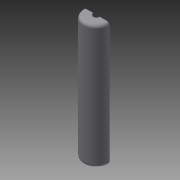
# Autodesk Inventor part: Wagon Hand Handle V04
Saved by Autodesk Inventor 2014 (Build 180170000, 170)
## iProperties
Created: 2013-11-30
Part Number: Wagon Hand Handle V04
Material: Generic
Document SubType Name: Modeling
Designer: steele
Density: 1 g/cm^3
Appearance: Default
Author: steele
Autodesk Inventor part; units mm, degrees
ref_plane "YZ Plane" through (0, 0, 0) normal (1, 0, 0) x (0, 1, 0)
ref_plane "XZ Plane" through (0, 0, 0) normal (0, 1, 0) x (-1, 0, 0)
ref_plane "XY Plane" through (0, 0, 0) normal (0, 0, 1) x (1, 0, 0)
sketch "Sketch1" plane through (0, 0, 0) normal (0, 0, 1) x (1, 0, 0)
  circle A0 centre (0, 0) radius 12.7
  circle A1 centre (0, 0) radius 3.302
  dimension "d0" = 25.4
  dimension "d1" = 6.604
  constraints: 2 centre point, 2 coincident
  measures "d0" diameter of A0
  measures "d1" diameter of A1
extrude "Extrusion1" add sketch "Sketch1" along normal mid plane 120.65
fillet "Fillet1" radius 3 2 edges at (-12.7, 0, 60.325) (-12.7, 0, -60.325)
sketch "Sketch3" plane through (0, 0, 60.325) normal (0, 0, 1) x (1, 0, 0)
  line L0 (-31, 0) -> (39, 0)
  line L1 (39, 0) -> (17, 30)
  line L2 (17, 30) -> (-16, 29)
  line L3 (-16, 29) -> (-31, 0)
  constraints: 8 end point, 1 horizontal
extrude "Extrusion2" cut sketch "Sketch3" against normal through all
sketch "Sketch4" plane through (-9.7, 0, 60.325) normal (0, 1, 0) x (1, 0, 0)
  line L0 (-3, 3) -> (-3, 117.65) projected
  line L1 (9.7, 0) -> (9.7, 120.65) construction
  circle A0 centre (9.7, 25.4) radius 8.8265
  circle A1 centre (9.7, 60.325) radius 8.8265
  circle A2 centre (9.7, 95.25) radius 8.8265
  circle A3 centre (9.7, 25.4) radius 5.7531
  circle A4 centre (9.7, 95.25) radius 5.7531
  circle A5 centre (9.7, 60.325) radius 5.7531
  line L2 (6.398, 120.65) -> (13.002, 120.65) projected
  dimension "d7" = 17.653
  dimension "d8" = 11.5062
  dimension "d16" = 60.325
  dimension "d17" = 25.4
  dimension "d18" = 25.4
  constraints: 6 centre point, 4 coincident, 4 equal radius, 2 end point, 2 point on line, 1 parallel
  measures "d7" diameter of A0
  measures "d8" diameter of A3
  measures "d16" distance of point (9.7, 60.325) L1.start
  measures "d17" distance of A0.centre L1.start
  measures "d18" distance from line of A2.centre L2
extrude "Extrusion3" cut sketch "Sketch4" against normal blind 9
sketch "Sketch7" plane through (-9.7, 0, 60.325) normal (0, 1, 0) x (1, 0, 0)
  line L0 (6.398, 52.1394) -> (6.398, 33.5856) projected
  line L1 (3.398, 34.5856) -> (3.398, 51.1394) construction
  line L2 (3.398, 34.2503) -> (3.398, 33.8516)
  line L3 (3.398, 33.8516) -> (1.9296, 33.8516)
  line L4 (1.9296, 33.8516) -> (1.9296, 32.4707)
  line L5 (1.9296, 32.4707) -> (3.398, 32.4707)
  line L6 (3.398, 32.4707) -> (3.398, 32.072)
  line L7 (3.398, 32.072) -> (0.398, 32.072)
  line L8 (0.398, 32.072) -> (0.398, 32.4707)
  line L9 (0.398, 32.4707) -> (1.5747, 32.4707)
  line L10 (1.5747, 32.4707) -> (1.5747, 33.8516)
  line L11 (1.5747, 33.8516) -> (0.398, 33.8516)
  line L12 (0.398, 33.8516) -> (0.398, 34.2503)
  line L13 (0.398, 34.2503) -> (3.398, 34.2503)
  spline S0 degree 2 poles (3.1598, 36.0833) (3.1938, 36.0371) (3.3153, 35.8815) (3.3518, 35.8086) knots 0 0 0 1 2 2 2
  spline S1 degree 2 poles (3.3518, 35.8086) (3.4053, 35.7089) (3.4612, 35.5217) (3.4612, 35.3516) knots 0 0 0 1 2 2 2
  spline S2 degree 2 poles (3.4612, 35.3516) (3.4612, 35.213) (3.3567, 34.9626) (3.2619, 34.8678) knots 0 0 0 1 2 2 2
  spline S3 degree 2 poles (3.2619, 34.8678) (3.1695, 34.7778) (2.8972, 34.6684) (2.7465, 34.6684) knots 0 0 0 1 2 2 2
  spline S4 degree 2 poles (2.7465, 34.6684) (2.5131, 34.6684) (2.1824, 34.8653) (2.0876, 35.0793) knots 0 0 0 1 2 2 2
  spline S5 degree 2 poles (2.0876, 35.0793) (2.0001, 35.2689) (1.9345, 35.7843) (1.9174, 36.0833) knots 0 0 0 1 2 2 2
  line L14 (1.9174, 36.0833) -> (1.8445, 36.0833)
  spline S6 degree 2 poles (1.8445, 36.0833) (1.7132, 36.0833) (1.5504, 36.0031) (1.5042, 35.9302) knots 0 0 0 1 2 2 2
  spline S7 degree 2 poles (1.5042, 35.9302) (1.458, 35.8572) (1.4288, 35.6482) (1.4288, 35.5363) knots 0 0 0 1 2 2 2
  spline S8 degree 2 poles (1.4288, 35.5363) (1.4288, 35.405) (1.5066, 35.0501) (1.582, 34.8726) knots 0 0 0 1 2 2 2
  line L15 (1.582, 34.8726) -> (1.582, 34.8507)
  line L16 (1.582, 34.8507) -> (1.1954, 34.8507)
  spline S9 degree 2 poles (1.1954, 34.8507) (1.1662, 34.9553) (1.0933, 35.3467) (1.0933, 35.5388) knots 0 0 0 1 2 2 2
  spline S10 degree 2 poles (1.0933, 35.5388) (1.0933, 35.7721) (1.1662, 36.0906) (1.261, 36.217) knots 0 0 0 1 2 2 2
  spline S11 degree 2 poles (1.261, 36.217) (1.3534, 36.341) (1.6476, 36.4626) (1.8591, 36.4626) knots 0 0 0 1 2 2 2
  line L17 (1.8591, 36.4626) -> (3.398, 36.4626)
  line L18 (3.398, 36.4626) -> (3.398, 36.0833)
  line L19 (3.398, 36.0833) -> (3.1598, 36.0833)
  line L20 (2.8437, 36.0833) -> (2.2189, 36.0833)
  spline S12 degree 2 poles (2.2189, 36.0833) (2.2311, 35.9472) (2.2724, 35.5363) (2.3113, 35.4075) knots 0 0 0 1 2 2 2
  spline S13 degree 2 poles (2.3113, 35.4075) (2.3575, 35.2567) (2.5495, 35.0598) (2.7197, 35.0598) knots 0 0 0 1 2 2 2
  spline S14 degree 2 poles (2.7197, 35.0598) (2.9142, 35.0598) (3.1111, 35.2786) (3.1111, 35.4877) knots 0 0 0 1 2 2 2
  spline S15 degree 2 poles (3.1111, 35.4877) (3.1111, 35.6652) (2.958, 35.9569) (2.8437, 36.0833) knots 0 0 0 1 2 2 2
  line L21 (3.398, 38.7624) -> (3.398, 38.3832)
  line L22 (3.398, 38.3832) -> (2.1144, 38.3832)
  spline S16 degree 2 poles (2.1144, 38.3832) (1.9588, 38.3832) (1.6914, 38.354) (1.6111, 38.3102) knots 0 0 0 1 2 2 2
  spline S17 degree 2 poles (1.6111, 38.3102) (1.526, 38.264) (1.4434, 38.0987) (1.4434, 37.9577) knots 0 0 0 1 2 2 2
  spline S18 degree 2 poles (1.4434, 37.9577) (1.4434, 37.8167) (1.5941, 37.5177) (1.7157, 37.3742) knots 0 0 0 1 2 2 2
  line L23 (1.7157, 37.3742) -> (3.398, 37.3742)
  line L24 (3.398, 37.3742) -> (3.398, 36.995)
  line L25 (3.398, 36.995) -> (1.1468, 36.995)
  line L26 (1.1468, 36.995) -> (1.1468, 37.3742)
  line L27 (1.1468, 37.3742) -> (1.3972, 37.3742)
  spline S19 degree 2 poles (1.3972, 37.3742) (1.244, 37.5444) (1.0836, 37.8726) (1.0836, 38.0574) knots 0 0 0 1 2 2 2
  spline S20 degree 2 poles (1.0836, 38.0574) (1.0836, 38.388) (1.5212, 38.7624) (1.9369, 38.7624) knots 0 0 0 1 2 2 2
  line L28 (1.9369, 38.7624) -> (3.398, 38.7624)
  line L29 (3.398, 41.0258) -> (3.398, 40.6465)
  line L30 (3.398, 40.6465) -> (3.1695, 40.6465)
  spline S21 degree 2 poles (3.1695, 40.6465) (3.2424, 40.559) (3.3397, 40.4302) (3.381, 40.3426) knots 0 0 0 1 2 2 2
  spline S22 degree 2 poles (3.381, 40.3426) (3.4199, 40.2624) (3.4612, 40.0898) (3.4612, 39.9755) knots 0 0 0 1 2 2 2
  spline S23 degree 2 poles (3.4612, 39.9755) (3.4612, 39.7908) (3.308, 39.4796) (3.1598, 39.3702) knots 0 0 0 1 2 2 2
  spline S24 degree 2 poles (3.1598, 39.3702) (3.0115, 39.2608) (2.5739, 39.1392) (2.2894, 39.1392) knots 0 0 0 1 2 2 2
  spline S25 degree 2 poles (2.2894, 39.1392) (1.9928, 39.1392) (1.5601, 39.2924) (1.3972, 39.4261) knots 0 0 0 1 2 2 2
  spline S26 degree 2 poles (1.3972, 39.4261) (1.2513, 39.5501) (1.0836, 39.8978) (1.0836, 40.0898) knots 0 0 0 1 2 2 2
  spline S27 degree 2 poles (1.0836, 40.0898) (1.0836, 40.2576) (1.1589, 40.508) (1.2367, 40.6465) knots 0 0 0 1 2 2 2
  line L31 (1.2367, 40.6465) -> (0.2643, 40.6465)
  line L32 (0.2643, 40.6465) -> (0.2643, 41.0258)
  line L33 (0.2643, 41.0258) -> (3.398, 41.0258)
  line L34 (2.851, 40.6465) -> (1.5504, 40.6465)
  spline S28 degree 2 poles (1.5504, 40.6465) (1.4823, 40.5055) (1.4312, 40.2819) (1.4312, 40.153) knots 0 0 0 1 2 2 2
  spline S29 degree 2 poles (1.4312, 40.153) (1.4312, 39.8613) (1.8688, 39.5307) (2.2821, 39.5307) knots 0 0 0 1 2 2 2
  spline S30 degree 2 poles (2.2821, 39.5307) (2.6808, 39.5307) (3.1014, 39.7835) (3.1014, 40.0631) knots 0 0 0 1 2 2 2
  spline S31 degree 2 poles (3.1014, 40.0631) (3.1014, 40.2114) (2.9653, 40.5128) (2.851, 40.6465) knots 0 0 0 1 2 2 2
  line L35 (3.398, 41.9618) -> (3.398, 41.5825)
  line L36 (3.398, 41.5825) -> (0.2643, 41.5825)
  line L37 (0.2643, 41.5825) -> (0.2643, 41.9618)
  line L38 (0.2643, 41.9618) -> (3.398, 41.9618)
  spline S32 degree 2 poles (3.4491, 43.4958) (3.4491, 42.9561) (2.8437, 42.3629) (2.2845, 42.3629) knots 0 0 0 1 2 2 2
  spline S33 degree 2 poles (2.2845, 42.3629) (1.7351, 42.3629) (1.0836, 42.9391) (1.0836, 43.4034) knots 0 0 0 1 2 2 2
  spline S34 degree 2 poles (1.0836, 43.4034) (1.0836, 43.6125) (1.2051, 43.9358) (1.334, 44.055) knots 0 0 0 1 2 2 2
  spline S35 degree 2 poles (1.334, 44.055) (1.4628, 44.1765) (1.8348, 44.3054) (2.1046, 44.3054) knots 0 0 0 1 2 2 2
  line L39 (2.1046, 44.3054) -> (2.3113, 44.3054)
  line L40 (2.3113, 44.3054) -> (2.3113, 42.747)
  spline S36 degree 2 poles (2.3113, 42.747) (2.7027, 42.747) (3.1184, 43.1409) (3.1184, 43.4909) knots 0 0 0 1 2 2 2
  spline S37 degree 2 poles (3.1184, 43.4909) (3.1184, 43.6149) (3.0625, 43.8556) (3.0187, 43.9529) knots 0 0 0 1 2 2 2
  spline S38 degree 2 poles (3.0187, 43.9529) (2.9701, 44.055) (2.885, 44.196) (2.8461, 44.2422) knots 0 0 0 1 2 2 2
  line L41 (2.8461, 44.2422) -> (2.8461, 44.264)
  line L42 (2.8461, 44.264) -> (3.2594, 44.264)
  spline S39 degree 2 poles (3.2594, 44.264) (3.2862, 44.1984) (3.364, 43.999) (3.3858, 43.9213) knots 0 0 0 1 2 2 2
  spline S40 degree 2 poles (3.3858, 43.9213) (3.4174, 43.8119) (3.4491, 43.6319) (3.4491, 43.4958) knots 0 0 0 1 2 2 2
  spline S41 degree 2 poles (2.022, 43.9358) (1.8688, 43.931) (1.6452, 43.8678) (1.5698, 43.807) knots 0 0 0 1 2 2 2
  spline S42 degree 2 poles (1.5698, 43.807) (1.4847, 43.7413) (1.3948, 43.5347) (1.3948, 43.3815) knots 0 0 0 1 2 2 2
  spline S43 degree 2 poles (1.3948, 43.3815) (1.3948, 43.2308) (1.4847, 43.0193) (1.5722, 42.9318) knots 0 0 0 1 2 2 2
  spline S44 degree 2 poles (1.5722, 42.9318) (1.6622, 42.8467) (1.8786, 42.7592) (2.022, 42.747) knots 0 0 0 1 2 2 2
  line L43 (2.022, 42.747) -> (2.022, 43.9358)
  line L44 (0.398, 48.183) -> (3.398, 47.1498)
  line L45 (3.398, 47.1498) -> (3.398, 46.7195)
  line L46 (3.398, 46.7195) -> (0.398, 45.6862)
  line L47 (0.398, 45.6862) -> (0.398, 46.1141)
  line L48 (0.398, 46.1141) -> (2.8899, 46.9456)
  line L49 (2.8899, 46.9456) -> (0.398, 47.777)
  line L50 (0.398, 47.777) -> (0.398, 48.183)
  spline S45 degree 2 poles (1.898, 51.5744) (2.7051, 51.5744) (3.4612, 51.1052) (3.4612, 50.6166) knots 0 0 0 1 2 2 2
  spline S46 degree 2 poles (3.4612, 50.6166) (3.4612, 50.1206) (2.6905, 49.6563) (1.9004, 49.6563) knots 0 0 0 1 2 2 2
  spline S47 degree 2 poles (1.9004, 49.6563) (1.0884, 49.6563) (0.3372, 50.1255) (0.3372, 50.6166) knots 0 0 0 1 2 2 2
  spline S48 degree 2 poles (0.3372, 50.6166) (0.3372, 51.1101) (1.1152, 51.5744) (1.898, 51.5744) knots 0 0 0 1 2 2 2
  spline S49 degree 2 poles (2.8121, 51.059) (2.6638, 51.1174) (2.2068, 51.166) (1.898, 51.166) knots 0 0 0 1 2 2 2
  spline S50 degree 2 poles (1.898, 51.166) (1.5892, 51.166) (1.1346, 51.1174) (0.9815, 51.0566) knots 0 0 0 1 2 2 2
  spline S51 degree 2 poles (0.9815, 51.0566) (0.8283, 50.9958) (0.6703, 50.7843) (0.6703, 50.6166) knots 0 0 0 1 2 2 2
  spline S52 degree 2 poles (0.6703, 50.6166) (0.6703, 50.4488) (0.8283, 50.2324) (0.9863, 50.1692) knots 0 0 0 1 2 2 2
  spline S53 degree 2 poles (0.9863, 50.1692) (1.1395, 50.1084) (1.6063, 50.0647) (1.9004, 50.0647) knots 0 0 0 1 2 2 2
  spline S54 degree 2 poles (1.9004, 50.0647) (2.2165, 50.0647) (2.6395, 50.1036) (2.8048, 50.1668) knots 0 0 0 1 2 2 2
  spline S55 degree 2 poles (2.8048, 50.1668) (2.9604, 50.2251) (3.1281, 50.4415) (3.1281, 50.6166) knots 0 0 0 1 2 2 2
  spline S56 degree 2 poles (3.1281, 50.6166) (3.1281, 50.7819) (2.9701, 50.9982) (2.8121, 51.059) knots 0 0 0 1 2 2 2
  line L51 (2.3672, 53.8888) -> (2.3672, 53.5315)
  line L52 (2.3672, 53.5315) -> (3.398, 53.5315)
  line L53 (3.398, 53.5315) -> (3.398, 53.1449)
  line L54 (3.398, 53.1449) -> (2.3672, 53.1449)
  line L55 (2.3672, 53.1449) -> (2.3672, 51.82)
  line L56 (2.3672, 51.82) -> (1.9442, 51.82)
  line L57 (1.9442, 51.82) -> (0.398, 53.1619)
  line L58 (0.398, 53.1619) -> (0.398, 53.5315)
  line L59 (0.398, 53.5315) -> (2.0439, 53.5315)
  line L60 (2.0439, 53.5315) -> (2.0439, 53.8888)
  line L61 (2.0439, 53.8888) -> (2.3672, 53.8888)
  line L62 (2.0439, 53.1449) -> (0.8721, 53.1449)
  line L63 (0.8721, 53.1449) -> (2.0439, 52.136)
  line L64 (2.0439, 52.136) -> (2.0439, 53.1449)
  dimension "d11" = 3
  dimension "d12" = 1
  dimension "d13" = 1
  constraints: 2 end point, 1 parallel, 1 vertical
  measures "d11" distance between parallel lines of L1 L0
  measures "d12" vertical distance of L1.start L0.end
  measures "d13" vertical distance of L0.start L1.end
emboss "Emboss1" sketch "Sketch7" operation cut depth 2 direction (0, -1, 0)
body "Solid1"
